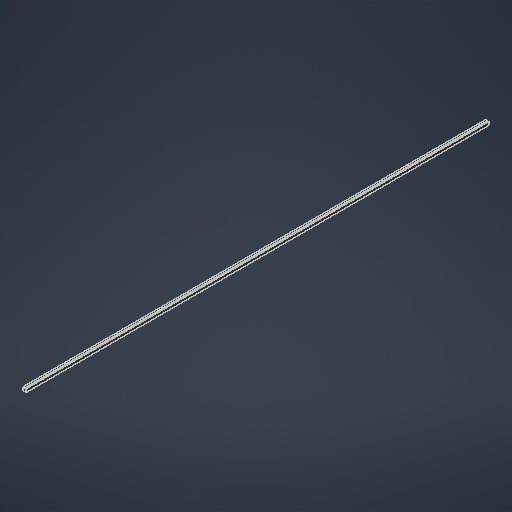
# Autodesk Inventor part: SP40-04A JUNTA INT CRISTAL ZOCALO 602 mm
Saved by Autodesk Inventor 2025 (Build 290162000, 162)
## iProperties
Created: 2026-01-20
Part Number: SP40-04A JUNTA INT CRISTAL ZOCALO 602 mm
Material: Caucho
Document SubType Name: Modeling
Designer: ROLANDO
Density: 0.93 g/cm^3
Appearance: Caucho - Negro
Author: ROLANDO
Autodesk Inventor part; units mm, degrees
ref_plane "YZ Plane" through (0, 0, 0) normal (1, 0, 0) x (0, 1, 0)
ref_plane "XZ Plane" through (0, 0, 0) normal (0, 1, 0) x (-1, 0, 0)
ref_plane "XY Plane" through (0, 0, 0) normal (0, 0, 1) x (1, 0, 0)
sketch "Boceto1" plane through (0, 0, 0) normal (0, 0, 1) x (1, 0, 0)
  line L0 (-0.9609, 42.0664) -> (-3.3609, 42.0664)
  line L1 (-3.3609, 42.0664) -> (-3.3609, 37.2556)
  line L2 (-0.9609, 42.0664) -> (-0.9609, 40.8164)
  line L3 (-0.9609, 40.8164) -> (-0.2551, 40.8164)
  line L4 (-0.2551, 40.8164) -> (0.4391, 41.8264)
  line L5 (-3.3609, 37.2556) -> (0.4391, 37.2556)
  line L6 (0.4391, 37.2556) -> (0.4391, 41.8264)
  constraints: 14 end point, 1 horizontal, 1 perpendicular
extrude "Extrusión1" add sketch "Boceto1" against normal blind 602
